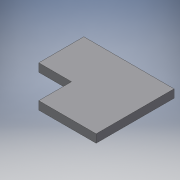
# Autodesk Inventor part: Supporto salita lama
Saved by Autodesk Inventor 2018 (Build 220112000, 112)
## iProperties
Created: 2020-06-16
Part Number: Supporto salita lama
Material: Generico
Document SubType Name: Modeling
Designer: Francesco
Density: 1 g/cm^3
Appearance: Acciaio - Lucido
Author: Francesco
Autodesk Inventor part; units mm, degrees
ref_plane "YZ Plane" through (0, 0, 0) normal (1, 0, 0) x (0, 1, 0)
ref_plane "XZ Plane" through (0, 0, 0) normal (0, 1, 0) x (-1, 0, 0)
ref_plane "XY Plane" through (0, 0, 0) normal (0, 0, 1) x (1, 0, 0)
sketch "Schizzo1" plane through (0, 0, 0) normal (0, 0, 1) x (1, 0, 0)
  line L0 (0, 0) -> (-40, 0)
  line L1 (-40, 0) -> (-40, 55)
  line L2 (-40, 55) -> (70, 55)
  line L3 (70, 55) -> (70, -40)
  line L4 (70, -40) -> (0, -40)
  line L5 (0, -40) -> (0, 0)
  dimension "d0" = 40
  dimension "d1" = 40
  dimension "d2" = 55
  dimension "d3" = 70
  constraints: 12 end point, 5 perpendicular, 1 horizontal
  measures "d0" distance between parallel lines of L4 L0
  measures "d1" distance between parallel lines of L1 L5
  measures "d2" distance between parallel lines of L2 L0
  measures "d3" distance between parallel lines of L5 L3
extrude "Estrusione1" add sketch "Schizzo1" along normal blind 10
fillet "Raccordo1" radius 5 5 edges at (-40, 55, 5) (70, 55, 5) (70, -40, 5) (-40, 0, 5) (0, -40, 5)
